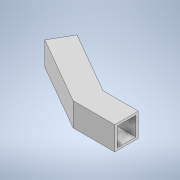
# Autodesk Inventor part: finger_one_bend_hollow
Saved by Autodesk Inventor 2021 (Build 250183000, 183)
## iProperties
Created: 2021-03-11
Part Number: finger_one_bend_hollow
Material: Generic
Document SubType Name: Modeling
Designer: Charlie
Density: 1 g/cm^3
Appearance: Default
Author: Charlie
Autodesk Inventor part; units mm, degrees
ref_plane "YZ Plane" through (0, 0, 0) normal (1, 0, 0) x (0, 1, 0)
ref_plane "XZ Plane" through (0, 0, 0) normal (0, 1, 0) x (-1, 0, 0)
ref_plane "XY Plane" through (0, 0, 0) normal (0, 0, 1) x (1, 0, 0)
sketch "Sketch1" plane through (0, 0, 0) normal (0, 1, 0) x (-1, 0, 0)
  line L0 (-15, 10) -> (20.359, 10)
  line L1 (25, 7.3205) -> (15, -10) construction
  line L2 (15, -10) -> (-15, -10)
  line L3 (-15, -10) -> (-15, 10)
  line L4 (-15, 10) -> (15, -10) construction
  line L5 (15, 10) -> (-15, -10) construction
  line L6 (20.359, 10) -> (50.9808, -7.6795)
  line L7 (50.9808, -7.6795) -> (40.9808, -25)
  line L8 (40.9808, -25) -> (15, -10)
  line L9 (15, -10) -> (15, 10) construction
  line L10 (50.9808, -7.6795) -> (76.9615, -22.6795)
  line L11 (76.9615, -22.6795) -> (66.9615, -40)
  line L12 (66.9615, -40) -> (40.9808, -25)
  line L13 (40.9808, -25) -> (50.9808, -7.6795)
  point P0 (0, 0)
  point P1 (15, -10)
  dimension "d0" = 30
  dimension "d3" = 30
  dimension "d4" = 20
  constraints: 28 end point, 4 parallel, 2 midpoint, 2 perpendicular, 2 point on line, 1 horizontal
  measures "d0" distance of L2.start L2.end
  measures "d3" distance of L11.end L12.end
  measures "d4" distance of L10.end L11.end
extrude "Extrusion1" add sketch "Sketch1" along normal blind 20
shell "Shell1" thickness 2 removed faces 2 at (15, 6.6667, 3.3333) at (-70.2949, 6.6667, -34.2265)
body "Solid1"
